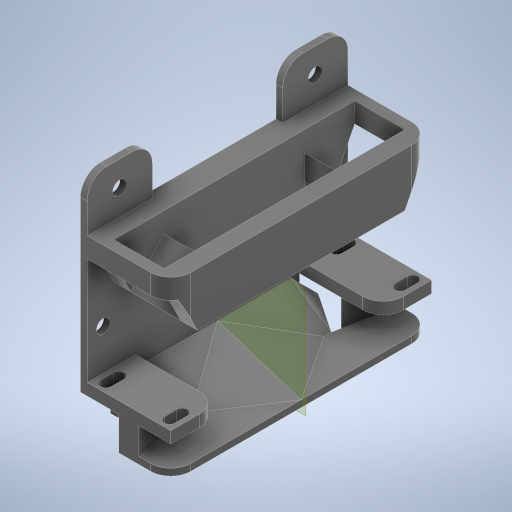
# Autodesk Inventor part: 12v_heater
Saved by Autodesk Inventor 2024 (Build 280153000, 153)
## iProperties
Created: 2024-10-17
Part Number: 12v_heater
Material: Acetal Resin, Black
Document SubType Name: Modeling
Designer: Owner
Density: 1.425 g/cm^3
Appearance: Smooth - Black
Author: Owner
Autodesk Inventor part; units mm, degrees
ref_plane "YZ Plane" through (0, 0, 0) normal (1, 0, 0) x (0, 1, 0)
ref_plane "XZ Plane" through (0, 0, 0) normal (0, 1, 0) x (-1, 0, 0)
ref_plane "XY Plane" through (0, 0, 0) normal (0, 0, 1) x (1, 0, 0)
sketch "Sketch1" plane through (0, 0, 0) normal (0, 1, 0) x (-1, 0, 0)
  line L0 (-15.875, 49.53) -> (15.875, 49.53)
  line L1 (15.875, 49.53) -> (15.875, -49.53)
  line L2 (15.875, -49.53) -> (-15.875, -49.53)
  line L3 (-15.875, -49.53) -> (-15.875, 49.53)
  line L4 (-15.875, 49.53) -> (15.875, -49.53) construction
  line L5 (15.875, 49.53) -> (-15.875, -49.53) construction
  line L6 (15.875, -49.53) -> (15.875, -48.26)
  line L7 (15.875, -49.53) -> (17.145, -49.53) construction
  line L8 (15.875, 49.53) -> (15.875, 48.26)
  line L9 (15.875, 49.53) -> (17.145, 49.53) construction
  line L10 (15.875, -49.53) -> (14.097, -49.53)
  line L11 (-15.875, -49.53) -> (-14.097, -49.53)
  line L12 (15.875, -49.53) -> (15.875, -39.37)
  line L13 (15.875, 49.53) -> (15.875, 39.37)
  line L14 (14.097, 49.53) -> (12.065, 49.53)
  line L15 (-14.097, 49.53) -> (-12.065, 49.53)
  line L16 (-12.065, -39.37) -> (-12.065, -48.26) construction
  line L17 (-10.033, -41.402) -> (-10.033, -46.228)
  line L18 (-14.097, -46.228) -> (-14.097, -41.402)
  arc A0 (-10.033, -41.402) -> (-14.097, -41.402) centre (-12.065, -41.402) ccw
  arc A1 (-14.097, -46.228) -> (-10.033, -46.228) centre (-12.065, -46.228) ccw
  line L19 (12.065, -48.26) -> (12.065, -39.37) construction
  line L20 (10.033, -46.228) -> (10.033, -41.402)
  line L21 (14.097, -41.402) -> (14.097, -46.228)
  arc A2 (10.033, -46.228) -> (14.097, -46.228) centre (12.065, -46.228) ccw
  arc A3 (14.097, -41.402) -> (10.033, -41.402) centre (12.065, -41.402) ccw
  line L22 (12.065, 39.37) -> (12.065, 48.26) construction
  line L23 (10.033, 41.402) -> (10.033, 46.228)
  line L24 (14.097, 46.228) -> (14.097, 41.402)
  arc A4 (10.033, 41.402) -> (14.097, 41.402) centre (12.065, 41.402) ccw
  arc A5 (14.097, 46.228) -> (10.033, 46.228) centre (12.065, 46.228) ccw
  line L25 (-12.065, 39.37) -> (-12.065, 48.26) construction
  line L26 (-10.033, 41.402) -> (-10.033, 46.228)
  line L27 (-14.097, 46.228) -> (-14.097, 41.402)
  arc A6 (-14.097, 41.402) -> (-10.033, 41.402) centre (-12.065, 41.402) ccw
  arc A7 (-10.033, 46.228) -> (-14.097, 46.228) centre (-12.065, 46.228) ccw
  line L28 (-12.065, 49.53) -> (-12.065, 37.6428)
  line L29 (-12.065, -37.6428) -> (-12.065, -49.53)
  line L30 (-14.097, -49.53) -> (-14.097, -39.37)
  line L31 (-14.097, 39.37) -> (-14.097, 49.53)
  line L32 (12.065, 49.53) -> (12.065, 37.6428)
  line L33 (12.065, -37.6428) -> (12.065, -49.53)
  line L34 (14.097, -49.53) -> (14.097, -39.37)
  line L35 (14.097, 39.37) -> (14.097, 49.53)
  line L36 (15.875, 39.37) -> (12.065, 39.37)
  line L37 (-12.065, 39.37) -> (-15.875, 39.37)
  line L38 (15.875, 48.26) -> (12.065, 48.26)
  line L39 (-12.065, 48.26) -> (-15.875, 48.26)
  line L40 (15.875, -39.37) -> (12.065, -39.37)
  line L41 (-12.065, -39.37) -> (-15.875, -39.37)
  line L42 (15.875, -48.26) -> (12.065, -48.26)
  line L43 (-12.065, -48.26) -> (-15.875, -48.26)
  point P0 (0, 0)
  point P1 (-12.065, -43.815)
  point P2 (12.065, -43.815)
  point P3 (12.065, 43.815)
  point P4 (-12.065, 43.815)
  dimension "d0" = 31.75
  dimension "d1" = 99.06
  dimension "d2" = 1.27
  dimension "d3" = 90
  dimension "d4" = 1.27
  dimension "d5" = 90
  dimension "d6" = 1.778
  dimension "d8" = 1.778
  dimension "d10" = 10.16
  dimension "d11" = 10.16
  dimension "d12" = 2.032
  dimension "d13" = 2.032
  constraints: 96 end point, 38 point on line, 24 point on circle, 16 tangent, 15 perpendicular, 8 centre point, 6 midpoint, 6 parallel, 3 horizontal, 2 collinear
  measures "d0" distance of L1.end L2.end
  measures "d1" distance of L0.end L1.end
  measures "d2" distance of L1.end L6.end
  measures "d3" angle of L7 L6
  measures "d4" distance of L0.end L8.end
  measures "d5" angle of L8 L9
  measures "d6" distance of L1.end L10.end
  measures "d8" distance of L2.end L11.end
  measures "d10" distance of L1.end L12.end
  measures "d11" distance of L0.end L13.end
  measures "d12" distance of L14.start L14.end
  measures "d13" distance of L15.start L15.end
extrude "Extrusion1" add sketch "Sketch1" along normal blind 4.445 contours L0 L31 L39 L3 | L0 L28 L39 L31 | L39 L31 L27 L37 L3 | L0 L32 A5 L23 A4 L36 L1 L40 A3 L20 A2 L33 L2 L29 A1 L17 A0 L41 L3 L37 A6 L26 A7 L28 | L39 A7 L31 | L0 L35 L38 L32 | L41 L30 L18 L43 L3 | L31 A6 L37 | L0 L1 L38 L35 | L38 L35 A5 | L43 L30 L2 L3 | L41 A0 L30 | L38 L1 L36 L35 L24 | A4 L35 L36 | L43 L29 L2 L30 | L30 A1 L43 | L1 L42 L34 L21 L40 | L33 L42 L34 L2 | L1 L2 L34 L42 | L34 A3 L40 | A2 L34 L42
sketch "Sketch2" plane through (0, 4.445, 0) normal (0, 1, 0) x (1, 0, 0)
  line L0 (15.875, -49.53) -> (15.875, 49.53) projected
  line L1 (-15.875, -31.115) -> (15.875, -31.115)
  line L2 (15.875, -31.115) -> (15.875, 31.115)
  line L3 (15.875, 31.115) -> (-15.875, 31.115)
  line L4 (-15.875, 31.115) -> (-15.875, -31.115)
  line L5 (-15.875, -31.115) -> (15.875, 31.115) construction
  line L6 (15.875, -31.115) -> (-15.875, 31.115) construction
  line L7 (-12.7, -31.115) -> (12.7, -31.115)
  line L8 (12.7, -31.115) -> (12.7, 31.115)
  line L9 (12.7, 31.115) -> (-12.7, 31.115)
  line L10 (-12.7, 31.115) -> (-12.7, -31.115)
  line L11 (-12.7, -31.115) -> (12.7, 31.115) construction
  line L12 (12.7, -31.115) -> (-12.7, 31.115) construction
  line L13 (-12.7, -26.67) -> (12.7, -26.67)
  line L14 (12.7, -26.67) -> (12.7, 26.67)
  line L15 (12.7, 26.67) -> (-12.7, 26.67)
  line L16 (-12.7, 26.67) -> (-12.7, -26.67)
  line L17 (-12.7, -26.67) -> (12.7, 26.67) construction
  line L18 (12.7, -26.67) -> (-12.7, 26.67) construction
  point P0 (0, 0)
  dimension "d16" = 62.23
  dimension "d19" = 25.4
  dimension "d20" = 53.34
  constraints: 36 end point, 6 midpoint, 6 parallel, 3 horizontal, 3 perpendicular, 3 point on line
  measures "d16" distance of L2.end L1.end
  measures "d19" distance of L9.end L8.end
  measures "d20" distance of L14.end L13.end
extrude "Extrusion2" cut sketch "Sketch2" against normal blind 4.445
sketch "Sketch7" plane through (0, 0, 0) normal (0, -1, 0) x (1, 0, 0)
  line L0 (-15.875, 31.115) -> (-15.875, 49.53) projected
  line L1 (-15.875, 49.53) -> (-18.415, 49.53)
  line L2 (-18.415, 49.53) -> (-18.415, -49.53)
  line L3 (-18.415, -49.53) -> (-15.875, -49.53)
  line L4 (-15.875, -49.53) -> (-15.875, 49.53)
  point P0 (0, 0)
  dimension "d34" = 2.54
  constraints: 8 end point, 2 parallel, 1 horizontal, 1 perpendicular
  measures "d34" distance of L3.end L2.end
extrude "Extrusion7" add sketch "Sketch7" along normal blind 12.7 and the other way blind 29.845
sketch "Sketch8" plane through (-15.875, 0, 49.53) normal (1, 0, 0) x (0, 0, -1)
  line L0 (99.06, -12.7) -> (0, -12.7) projected
  line L1 (99.06, 29.845) -> (99.06, -12.7) projected
  line L2 (0, -12.7) -> (99.06, -12.7)
  line L3 (99.06, -12.7) -> (99.06, -10.16)
  line L4 (99.06, -10.16) -> (0, -10.16)
  line L5 (0, -10.16) -> (0, -12.7)
  point P0 (49.53, 0)
  dimension "d39" = 2.54
  constraints: 8 end point, 2 parallel, 1 horizontal, 1 perpendicular, 1 point on line
  measures "d39" distance of L3.end L2.end
extrude "Extrusion8" add sketch "Sketch8" along normal blind 31.75
ref_plane "Work Plane1" through (15.875, 0, 0) normal (0, 0, -1) x (-1, 0, 0)
sketch "Sketch10" plane through (15.875, 0, 0) normal (0, 0, -1) x (-1, 0, 0)
  line L0 (0, 0) -> (31.75, 0) projected
  line L1 (31.75, -10.16) -> (0, -10.16) projected
  line L2 (31.75, 0) -> (0, -10.16)
  line L3 (0, -10.16) -> (31.75, -10.16)
  line L4 (31.75, -10.16) -> (31.75, 0)
  point P0 (15.875, 0)
  constraints: 6 end point, 1 collinear, 1 perpendicular
extrude "Extrusion10" add sketch "Sketch10" along normal mid plane 63.5
chamfer "Chamfer3" distance 6.35 distance2 31.75 1 edges at (0, -5.08, 31.75) measured on face at (-0.1524, -5.5562, 31.75)
chamfer "Chamfer4" distance 6.35 distance2 31.75 1 edges at (0, -5.08, -31.75) measured on face at (-0.1524, -5.5562, -31.75)
sketch "Sketch11" plane through (15.875, 0, 0) normal (0, 0, -1) x (-1, 0, 0)
  line L0 (31.75, -10.16) -> (31.75, 0) projected
  line L1 (31.75, 0) -> (31.75, -10.16)
  line L2 (31.75, -10.16) -> (16.51, -10.16)
  line L3 (16.51, -10.16) -> (31.75, 0)
  point P0 (15.875, 0)
  dimension "d59" = 15.24
  constraints: 6 end point, 1 collinear, 1 perpendicular
  measures "d59" distance of L0.start L2.end
extrude "Extrusion11" add sketch "Sketch11" along normal mid plane 76.2
chamfer "Chamfer5" distance 8.382 distance2 10.16 1 edges at (-8.255, -5.08, 38.1) measured on face at (-8.5324, -5.496, 38.1)
chamfer "Chamfer6" distance 8.382 distance2 10.16 1 edges at (-8.255, -5.08, -38.1) measured on face at (-8.5324, -5.496, -38.1)
sketch "Sketch12" plane through (-15.875, 0, -31.115) normal (1, 0, 0) x (0, 0, -1)
  line L0 (-62.23, 0) -> (-80.645, 0) projected
  line L1 (-62.23, 0) -> (-62.23, -3.1481)
  line L2 (-59.055, 0) -> (-69.215, -10.0739) projected
  line L3 (-80.645, -10.16) -> (-69.215, -10.16) projected
  line L4 (-62.23, -3.1481) -> (-69.215, -10.16)
  line L5 (-69.215, -10.16) -> (-80.645, -10.16)
  line L6 (-80.645, 0) -> (-80.645, -10.16) projected
  line L7 (-80.645, -10.16) -> (-80.645, 0)
  line L8 (-80.645, 0) -> (-62.23, 0)
  line L9 (0, 4.445) -> (0, 0) projected
  line L10 (0, 0) -> (0, -3.1481)
  line L11 (-3.175, 0) -> (6.985, -10.0739) projected
  line L12 (0, -3.1481) -> (11.7987, -14.8468)
  line L13 (18.415, -10.16) -> (-31.115, -10.16) projected
  line L14 (7.0718, -10.16) -> (18.415, -10.16)
  line L15 (0, 0) -> (18.415, 0) projected
  line L16 (18.415, -10.16) -> (18.415, 0)
  line L17 (18.415, 0) -> (0, 0)
  point P0 (-31.115, 0)
  constraints: 20 end point, 4 collinear, 4 point on line, 3 perpendicular, 1 vertical
extrude "Extrusion12" cut sketch "Sketch12" against normal blind 76.2
sketch "Sketch13" plane through (0, 0, 0) normal (0, -1, 0) x (1, 0, 0)
  line L0 (-18.415, 49.53) -> (15.875, 49.53) projected
  line L1 (0, 49.53) -> (3.81, 49.53)
  line L2 (3.81, 49.53) -> (-3.81, 49.53)
  line L3 (-3.81, 49.53) -> (0, 31.115)
  line L4 (-15.875, 31.115) -> (15.875, 31.115) projected
  line L5 (3.81, 49.53) -> (0, 31.115)
  line L6 (15.875, -49.53) -> (-18.415, -49.53) projected
  line L7 (0, -49.53) -> (-3.81, -49.53)
  line L8 (0, -49.53) -> (3.81, -49.53)
  line L9 (3.81, -49.53) -> (0, -31.115)
  line L10 (15.875, -31.115) -> (-15.875, -31.115) projected
  line L11 (-3.81, -49.53) -> (0, -31.115)
  point P0 (0, 0)
  dimension "d70" = 3.81
  dimension "d71" = 7.62
  constraints: 16 end point, 6 point on line, 2 midpoint, 1 parallel
  measures "d70" distance of L1.start L1.end
  measures "d71" distance of L1.end L2.end
extrude "Extrusion13" add sketch "Sketch13" along normal blind 10.16
sketch "Sketch14" plane through (0, 29.845, 0) normal (0, 1, 0) x (1, 0, 0)
  line L0 (-18.415, 49.53) -> (-18.415, 31.115) projected
  line L1 (-15.875, -49.53) -> (-15.875, 49.53) projected
  line L2 (-18.415, 49.53) -> (-15.875, 49.53)
  line L3 (-15.875, 49.53) -> (-15.875, -49.53)
  line L4 (-15.875, -49.53) -> (-18.415, -49.53)
  line L5 (-18.415, -49.53) -> (-18.415, 49.53)
  point P0 (0, 0)
  constraints: 8 end point, 2 parallel, 1 horizontal, 1 perpendicular
extrude "Extrusion14" add sketch "Sketch14" along normal blind 15.24
sketch "Sketch15" plane through (0, 45.085, 0) normal (0, 1, 0) x (1, 0, 0)
  line L0 (-9.525, -45.72) -> (9.525, -45.72)
  line L1 (9.525, -45.72) -> (9.525, 45.72)
  line L2 (9.525, 45.72) -> (-9.525, 45.72)
  line L3 (-9.525, 45.72) -> (-9.525, -45.72)
  line L4 (-9.525, -45.72) -> (9.525, 45.72) construction
  line L5 (9.525, -45.72) -> (-9.525, 45.72) construction
  line L6 (-18.415, -49.53) -> (-18.415, -38.1) projected
  line L7 (15.875, 49.53) -> (-15.875, 49.53) projected
  line L8 (-18.415, -49.53) -> (-15.875, -49.53)
  line L9 (-15.875, -49.53) -> (-15.875, 49.53)
  line L10 (-15.875, 49.53) -> (-18.415, 49.53)
  line L11 (-18.415, 49.53) -> (-18.415, -49.53)
  line L12 (-15.875, -49.53) -> (15.875, -49.53)
  line L13 (15.875, -49.53) -> (15.875, 49.53)
  line L14 (-15.875, -49.53) -> (-15.875, 49.53) projected
  line L15 (-15.875, 49.53) -> (15.875, 49.53)
  point P0 (0, 0)
  dimension "d76" = 19.05
  dimension "d77" = 91.44
  constraints: 26 end point, 5 parallel, 3 horizontal, 2 midpoint, 2 perpendicular, 1 collinear
  measures "d76" distance of L2.end L1.end
  measures "d77" distance of L1.end L0.end
extrude "Extrusion15" add sketch "Sketch15" along normal blind 7.62
sketch "Sketch16" plane through (-15.875, 4.445, -31.115) normal (1, 0, 0) x (0, 0, -1)
  line L0 (14.605, 40.64) -> (-76.835, 40.64) projected
  line L1 (-31.115, 40.64) -> (-57.785, 40.64)
  line L2 (-57.785, 40.64) -> (-4.445, 40.64)
  line L3 (-4.445, 40.64) -> (-4.445, 27.94)
  line L4 (-4.445, 27.94) -> (8.255, 27.94)
  line L5 (8.255, 27.94) -> (-4.445, 40.64)
  line L6 (-57.785, 40.64) -> (-57.785, 27.94)
  line L7 (-57.785, 27.94) -> (-70.485, 27.94)
  line L8 (-70.485, 27.94) -> (-57.785, 40.64)
  point P0 (-31.115, -4.445)
  dimension "d80" = 26.67
  dimension "d81" = 53.34
  dimension "d82" = 12.7
  dimension "d83" = 12.7
  dimension "d84" = 12.7
  dimension "d85" = 12.7
  constraints: 16 end point, 5 point on line, 3 perpendicular, 1 midpoint
  measures "d80" distance of L1.start L1.end
  measures "d81" distance of L1.end L2.end
  measures "d82" distance of L2.end L3.end
  measures "d83" distance of L3.end L4.end
  measures "d84" distance of L1.end L6.end
  measures "d85" distance of L6.end L7.end
extrude "Extrusion16" add sketch "Sketch16" along normal up to surface (25.4 mm away)
fillet "Fillet1" radius 3.175 2 edges at (-3.175, 32.385, 26.67) (-3.175, 32.385, -26.67)
sketch "Sketch17" plane through (0, 45.085, 0) normal (0, -1, 0) x (1, 0, 0)
  line L0 (15.875, -49.53) -> (-18.415, -49.53) projected
  line L1 (15.875, -49.53) -> (-15.875, -49.53)
  line L2 (-15.875, -49.53) -> (-15.875, 49.53)
  line L3 (-15.875, 49.53) -> (15.875, 49.53)
  line L4 (15.875, 49.53) -> (15.875, -49.53)
  line L5 (-9.525, -26.67) -> (-9.525, -45.72) projected
  line L6 (9.525, 45.72) -> (-9.525, 45.72)
  line L7 (-9.525, 45.72) -> (-9.525, -45.72)
  line L8 (-9.525, -45.72) -> (9.525, -45.72)
  line L9 (9.525, -45.72) -> (9.525, 45.72)
  line L10 (-9.525, 45.72) -> (-15.875, 45.72)
  line L11 (9.525, 45.72) -> (15.875, 45.72)
  line L12 (-9.525, -45.72) -> (-15.875, -45.72)
  line L13 (9.525, -45.72) -> (15.875, -45.72)
  point P0 (0, 0)
  constraints: 24 end point, 7 point on line, 4 parallel, 3 perpendicular, 2 horizontal
extrude "Extrusion17" add sketch "Sketch17" along normal blind 12.7 contours L13 L9 L11 L4 | L2 L10 L7 L5 L12
chamfer "Chamfer7" distance 6.35 distance2 12.7 4 edges at (12.7, 32.385, -45.72) (12.7, 32.385, 45.72) (-12.7, 32.385, -45.72) (-12.7, 32.385, 45.72) measured on face at (12.7, 32.385, 45.22) measured on face at (-12.7, 32.385, -45.22) measured on face at (12.7, 32.385, -45.22) measured on face at (-12.7, 32.385, 45.22)
sketch "Sketch18" plane through (0, 52.705, 0) normal (0, 1, 0) x (1, 0, 0)
  line L0 (-18.415, -31.115) -> (-18.415, -49.53) projected
  line L1 (-15.875, 49.53) -> (-15.875, 31.115) projected
  line L2 (-18.415, -49.53) -> (-15.875, -49.53)
  line L3 (-15.875, -49.53) -> (-15.875, 49.53)
  line L4 (-15.875, 49.53) -> (-18.415, 49.53)
  line L5 (-18.415, 49.53) -> (-18.415, -49.53)
  point P0 (0, 0)
  constraints: 8 end point, 2 parallel, 1 horizontal, 1 perpendicular
extrude "Extrusion18" add sketch "Sketch18" along normal blind 19.05
sketch "Sketch19" plane through (-15.875, 52.705, 49.53) normal (1, 0, 0) x (0, 0, -1)
  line L0 (0, 0) -> (0, 19.05) projected
  line L1 (99.06, 19.05) -> (99.06, -52.705) projected
  line L2 (0, 0) -> (99.06, 0)
  line L3 (99.06, 0) -> (99.06, 19.05)
  line L4 (99.06, 19.05) -> (0, 19.05)
  line L5 (0, 19.05) -> (0, 0)
  line L6 (0, 9.525) -> (99.06, 9.525)
  line L7 (99.06, 19.05) -> (0, 19.05) projected
  line L8 (49.53, 19.05) -> (49.53, 0)
  line L9 (0, 19.05) -> (49.53, 19.05)
  line L10 (49.53, 19.05) -> (49.53, 0)
  line L11 (49.53, 0) -> (0, 0)
  line L12 (0, 0) -> (0, 19.05)
  line L13 (99.06, 19.05) -> (49.53, 19.05)
  line L14 (49.53, 19.05) -> (49.53, 0)
  line L15 (49.53, 0) -> (99.06, 0)
  line L16 (99.06, 0) -> (99.06, 19.05)
  line L17 (95.25, 0) -> (3.81, 0) projected
  line L18 (0, 19.05) -> (24.765, 19.05)
  line L19 (24.765, 19.05) -> (24.765, 0)
  line L20 (24.765, 0) -> (0, 0)
  line L21 (0, 0) -> (0, 19.05)
  line L22 (99.06, 19.05) -> (74.295, 19.05)
  line L23 (74.295, 19.05) -> (74.295, 0)
  line L24 (74.295, 0) -> (99.06, 0)
  line L25 (99.06, 0) -> (99.06, 19.05)
  line L26 (99.06, 19.05) -> (86.6775, 19.05)
  line L27 (86.6775, 19.05) -> (86.6775, 0)
  line L28 (86.6775, 0) -> (99.06, 0)
  line L29 (99.06, 0) -> (99.06, 19.05)
  line L30 (0, 19.05) -> (12.3825, 19.05)
  line L31 (12.3825, 19.05) -> (12.3825, 0)
  line L32 (12.3825, 0) -> (0, 0)
  line L33 (0, 0) -> (0, 19.05)
  circle A0 centre (12.3825, 9.525) radius 2.667
  circle A1 centre (86.6775, 9.525) radius 2.667
  line L34 (12.3825, 19.05) -> (12.3825, -66.0843)
  line L35 (86.6775, 19.05) -> (86.6775, -70.5342)
  line L36 (0, -48.26) -> (18.415, -48.26) projected
  line L37 (0, -48.26) -> (99.06, -48.26)
  line L38 (99.06, -48.26) -> (99.06, -7.3323)
  line L39 (99.06, -7.3323) -> (0, -7.3323)
  line L40 (0, -7.3323) -> (0, -48.26)
  line L41 (6.1912, 19.05) -> (6.1912, -48.26)
  line L42 (92.8688, 19.05) -> (92.8688, -48.26)
  line L43 (0, -27.7962) -> (99.06, -27.7962)
  line L44 (0, -27.7962) -> (0, -37.9562)
  line L45 (0, -37.9562) -> (99.06, -37.9562)
  line L46 (0, -32.8762) -> (99.06, -32.8762)
  circle A2 centre (6.1912, -32.8762) radius 2.667
  circle A3 centre (92.8688, -32.8762) radius 2.667
  point P0 (49.53, -52.705)
  dimension "d96" = 5.334
  dimension "d97" = 5.334
  dimension "d98" = 10.16
  dimension "d99" = 5.334
  dimension "d100" = 5.334
  constraints: 84 end point, 18 parallel, 14 midpoint, 12 point on line, 10 perpendicular, 8 horizontal, 4 centre point, 1 vertical
  measures "d96" diameter of A0
  measures "d97" diameter of A1
  measures "d98" distance of L43.start L44.end
  measures "d99" diameter of A2
  measures "d100" diameter of A3
extrude "Extrusion19" cut sketch "Sketch19" against normal blind 19.05 contours A0 L31 L6 | L6 L31 A0 | L31 A0 L6 | L6 A0 L31 | A2 L46 L41 | L41 L46 A2 | L46 A2 L41 | L41 A2 L46 | A1 L6 L27 | L27 L6 A1 | A1 L27 L6 | A3 L42 L46 | L46 L42 A3 | A3 L46 L42 | L27 A1 L6 | L46 A3 L42
fillet "Fillet2" radius 7.62 2 edges at (-17.145, 71.755, 49.53) (-17.145, 71.755, -49.53)
sketch "Sketch20" plane through (0, -12.7, 0) normal (0, -1, 0) x (1, 0, 0)
  line L0 (-0.635, -27.94) -> (-15.7459, -38.1) projected
  line L1 (-18.415, -49.53) -> (-15.7459, -49.53)
  line L2 (-15.7459, -49.53) -> (-15.7459, -38.1)
  line L3 (-15.7459, -38.1) -> (-18.415, -38.1)
  line L4 (-18.415, -38.1) -> (-18.415, -49.53)
  line L5 (-15.7459, -38.1) -> (-0.635, -27.94)
  line L6 (-3.81, -49.53) -> (0, -31.115) projected
  line L7 (-3.81, -49.53) -> (0, -31.115)
  line L8 (0, -31.115) -> (-0.635, -27.94)
  line L9 (-3.81, -49.53) -> (-15.7459, -49.53)
  line L10 (-18.415, 49.53) -> (-18.415, -49.53) projected
  line L11 (-18.415, -38.1) -> (-18.415, -38.1)
  line L12 (-18.415, -38.1) -> (-18.415, -49.53)
  line L13 (-18.415, -49.53) -> (-18.415, -49.53)
  line L14 (-18.415, -49.53) -> (-18.415, -38.1)
  line L15 (-15.7459, 38.1) -> (-0.635, 27.94) projected
  line L16 (-15.7459, 38.1) -> (-18.415, 38.1)
  line L17 (-18.415, 38.1) -> (-18.415, 49.5634)
  line L18 (-18.415, 49.5634) -> (-15.7459, 49.5634)
  line L19 (-15.7459, 49.5634) -> (-15.7459, 38.1)
  line L20 (-0.635, 27.94) -> (-15.875, 27.94) projected
  line L21 (-15.7459, 38.1) -> (-0.635, 27.94)
  line L22 (0, 31.115) -> (3.81, 49.53) projected
  line L23 (-0.635, 27.94) -> (0, 31.115)
  line L24 (0, 31.115) -> (-3.81, 49.53) projected
  line L25 (0, 31.115) -> (-3.81, 49.53)
  line L26 (-3.81, 49.53) -> (-15.7459, 49.5634)
  point P0 (0, 0)
  constraints: 40 end point, 9 equal length, 4 horizontal, 3 perpendicular, 2 point on line
extrude "Extrusion20" cut sketch "Sketch20" against normal blind 2.54
fillet "Fillet3" radius 7.62 4 edges at (15.875, 2.2225, -31.115) (15.875, 2.2225, 31.115) (15.875, -11.43, -49.53) (15.875, -11.43, 49.53)
fillet "Fillet4" radius 7.62 2 edges at (15.875, 48.895, 49.53) (15.875, 48.895, -49.53)
sketch "Sketch21" plane through (-15.875, 52.705, 49.53) normal (1, 0, 0) x (0, 0, -1)
  line L0 (24.765, 0) -> (0, 0)
  line L1 (0, 0) -> (0, 19.05)
  line L2 (0, 19.05) -> (24.765, 19.05)
  line L3 (24.765, 19.05) -> (24.765, 0)
  circle A0 centre (12.3825, 9.525) radius 2.667 projected
  line L4 (24.765, 0) -> (0, 19.05) construction
  line L5 (0, 0) -> (24.765, 19.05) construction
  line L6 (74.295, 0) -> (99.06, 0)
  line L7 (99.06, 0) -> (99.06, 19.05)
  line L8 (99.06, 19.05) -> (74.295, 19.05)
  line L9 (74.295, 19.05) -> (74.295, 0)
  circle A1 centre (86.6775, 9.525) radius 2.667 projected
  line L10 (74.295, 0) -> (99.06, 19.05) construction
  line L11 (99.06, 0) -> (74.295, 19.05) construction
  line L12 (24.765, 19.05) -> (74.295, 19.05)
  line L13 (74.295, 19.05) -> (74.295, 0)
  line L14 (74.295, 0) -> (24.765, 0)
  line L15 (24.765, 0) -> (24.765, 19.05)
  point P0 (49.53, -52.705)
  point P1 (74.295, 19.05)
  point P2 (24.765, 0)
  constraints: 32 end point, 6 parallel, 4 midpoint, 3 horizontal, 3 perpendicular, 1 point on line
extrude "Extrusion21" cut sketch "Sketch21" against normal blind 2.54 contours L3 L12 L9 L14
fillet "Fillet5" radius 7.62 2 edges at (-17.145, 71.755, -24.765) (-17.145, 71.755, 24.765)
equation "\"d17\" = d14"
equation "\"d14\" = 4.445"
body "Solid1"
